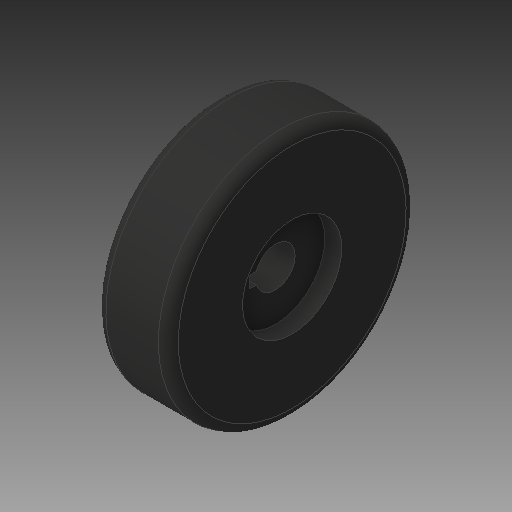
# Autodesk Inventor part: 100mm Traction Wheel StandIn
Saved by Autodesk Inventor 2019.4 (Build 234330000, 330)
## iProperties
Created: 2019-10-18
Part Number: 100mm Traction Wheel StandIn
Material: Rubber
Document SubType Name: Modeling
Designer: admin
Density: 0.93 g/cm^3
Appearance: Rubber - Black
Author: admin
Autodesk Inventor part; units mm, degrees
ref_plane "YZ Plane" through (0, 0, 0) normal (1, 0, 0) x (0, 1, 0)
ref_plane "XZ Plane" through (0, 0, 0) normal (0, 1, 0) x (-1, 0, 0)
ref_plane "XY Plane" through (0, 0, 0) normal (0, 0, 1) x (1, 0, 0)
sketch "Sketch1" plane through (0, 0, 0) normal (1, 0, 0) x (0, 1, 0)
  circle A0 centre (0, 0) radius 62.5
  dimension "d0" = 125
  constraints: 1 centre point, 1 coincident
  measures "d0" diameter of A0
extrude "Extrusion1" add sketch "Sketch1" along normal blind 36.5
fillet "Fillet1" radius 5 2 edges at (36.5, -62.5, 0) (0, -62.5, 0)
sketch "Sketch2" plane through (36.5, 0, 0) normal (1, 0, 0) x (0, 0, -1)
  circle A0 centre (0, 0) radius 62.5 projected
  constraints: 1 coincident
hole "Hole1" at (36.5, 0, 0) direction (-1, 0, 0) diameter 20 end through all
sketch "Sketch3" plane through (36.5, 0, 0) normal (1, 0, 0) x (0, 0, -1)
  circle A0 centre (0, 0) radius 25
  dimension "d11" = 50
  constraints: 1 centre point, 1 coincident
  measures "d11" diameter of A0
extrude "Extrusion2" cut sketch "Sketch3" against normal blind 8.5
sketch "Sketch4" plane through (28, 0, 0) normal (1, 0, 0) x (0, 0, -1)
  line L0 (-7, -3) -> (-13, -3)
  line L1 (-13, -3) -> (-13, 3)
  line L2 (-13, 3) -> (-7, 3)
  line L3 (-7, 3) -> (-7, -3)
  circle A0 centre (0, 0) radius 10 projected
  line L4 (-7, -3) -> (-13, 3) construction
  line L5 (-13, -3) -> (-7, 3) construction
  point P0 (-10, 0)
  dimension "d14" = 6
  dimension "d15" = 6
  constraints: 12 end point, 2 midpoint, 2 parallel, 1 horizontal, 1 horizontal alignment, 1 perpendicular, 1 other
  measures "d14" distance of L1.end L2.end
  measures "d15" distance of L0.end L1.end
extrude "Extrusion3" cut sketch "Sketch4" against normal blind 28 contours L0 A0 L2 L3 | L0 L1 L2 A0 picked at (-7.9828, 0.338)
body "Solid1"
